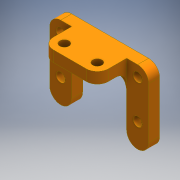
# Autodesk Inventor part: cam_holder
Saved by Autodesk Inventor 2016 (Build 200138000, 138)
## iProperties
Created: 2016-09-23
Part Number: cam_holder
Material: Nylon 6/6
Document SubType Name: Modeling
Designer: Jakub
Density: 1.13 g/cm^3
Appearance: Nylon 6
Author: Jakub
Autodesk Inventor part; units mm, degrees
ref_plane "YZ Plane" through (0, 0, 0) normal (1, 0, 0) x (0, 1, 0)
ref_plane "XZ Plane" through (0, 0, 0) normal (0, 1, 0) x (-1, 0, 0)
ref_plane "XY Plane" through (0, 0, 0) normal (0, 0, 1) x (1, 0, 0)
sketch "Sketch1" plane through (0, 0, 0) normal (0, 1, 0) x (-1, 0, 0)
  line L0 (13.5, 10) -> (-13.5, 10)
  line L1 (-13.5, 10) -> (-13.5, -10)
  line L2 (-13.5, -10) -> (13.5, -10)
  line L3 (13.5, -10) -> (13.5, 10)
  line L4 (13.5, 10) -> (-13.5, -10) construction
  line L5 (-13.5, 10) -> (13.5, -10) construction
  point P0 (0, 0)
  dimension "d0" = 27
  dimension "d1" = 20
  constraints: 12 end point, 2 midpoint, 2 parallel, 1 horizontal, 1 perpendicular
  measures "d0" distance of L2.end L1.end
  measures "d1" distance of L1.end L0.end
extrude "Extrusion1" add sketch "Sketch1" along normal blind 3
sketch "Sketch2" plane through (0, 3, 0) normal (0, 1, 0) x (1, 0, 0)
  line L0 (-13.5, -10) -> (13.5, -10) projected
  line L1 (0, -10) -> (-10.5, -10)
  line L2 (-10.5, -10) -> (-10.5, -7)
  line L3 (-10.5, -7) -> (-10.5, 3.5)
  circle A0 centre (-10.5, -7) radius 1.25
  circle A1 centre (-10.5, 3.5) radius 1.25
  line L4 (-10.5, -7) -> (10.5, -7)
  line L5 (10.5, -7) -> (10.5, 3.5)
  circle A2 centre (10.5, -7) radius 1.25
  circle A3 centre (10.5, 3.5) radius 1.25
  point P0 (0, 0)
  dimension "d4" = 10.5
  dimension "d5" = 3
  dimension "d6" = 10.5
  dimension "d7" = 2.5
  dimension "d8" = 2.5
  dimension "d9" = 21
  dimension "d10" = 10.5
  dimension "d11" = 2.5
  dimension "d12" = 2.5
  constraints: 10 end point, 4 centre point, 4 coincident, 2 point on line, 1 horizontal, 1 midpoint, 1 perpendicular, 1 vertical
  measures "d4" distance of L1.start L1.end
  measures "d5" distance of L1.end L2.end
  measures "d6" distance of L2.end L3.end
  measures "d7" diameter of A0
  measures "d8" diameter of A1
  measures "d9" distance of L4.start L4.end
  measures "d10" distance of L4.end L5.end
  measures "d11" diameter of A2
  measures "d12" diameter of A3
extrude "Extrusion2" cut sketch "Sketch2" against normal up to next
sketch "Sketch3" plane through (0, 0, 0) normal (0, -1, 0) x (1, 0, 0)
  line L0 (-13.5, 10) -> (13.5, 10) projected
  line L1 (0, 10) -> (0, 8.5)
  line L2 (7.5, 7) -> (-7.5, 7)
  line L3 (-7.5, 7) -> (-7.5, 10)
  line L4 (-7.5, 10) -> (7.5, 10)
  line L5 (7.5, 10) -> (7.5, 7)
  line L6 (7.5, 7) -> (-7.5, 10) construction
  line L7 (-7.5, 7) -> (7.5, 10) construction
  point P0 (0, 0)
  dimension "d15" = 1.5
  dimension "d16" = 15
  dimension "d17" = 3
  constraints: 14 end point, 3 midpoint, 2 parallel, 1 horizontal, 1 perpendicular, 1 vertical
  measures "d15" distance of L1.start L1.end
  measures "d16" distance of L3.end L4.end
  measures "d17" distance of L2.end L3.end
extrude "Extrusion3" add sketch "Sketch3" along normal blind 8
sketch "Sketch4" plane through (7.5, 0, 7) normal (0, 0, -1) x (-1, 0, 0)
  circle A0 centre (3, -5) radius 1.25
  circle A1 centre (12, -5) radius 1.25
  line L0 (0, 0) -> (0, -8) projected
  line L1 (15, -8) -> (0, -8) projected
  line L2 (15, 0) -> (15, -8) projected
  point P0 (7.5, 0)
  dimension "d20" = 2.5
  dimension "d21" = 2.5
  dimension "d22" = 3
  dimension "d23" = 3
  dimension "d24" = 3
  dimension "d25" = 3
  constraints: 2 centre point
  measures "d20" diameter of A0
  measures "d21" diameter of A1
  measures "d22" distance from line of L0 A0.centre
  measures "d23" distance from line of L1 A0.centre
  measures "d24" distance from line of L2 A1.centre
  measures "d25" distance from line of L1 A1.centre
extrude "Extrusion4" cut sketch "Sketch4" against normal up to next
sketch "Sketch5" plane through (0, 0, 0) normal (0, -1, 0) x (1, 0, 0)
  line L0 (13.5, -10) -> (-13.5, -10) projected
  line L1 (13.5, -10) -> (7.5, -10)
  line L2 (7.5, -10) -> (-7.5, -10)
  line L3 (-7.5, -10) -> (-7.5, 7)
  line L4 (-7.5, 7) -> (7.5, 7)
  line L5 (7.5, 7) -> (7.5, -10)
  point P0 (0, 0)
  dimension "d28" = 6
  constraints: 10 end point, 2 parallel, 1 horizontal, 1 perpendicular, 1 point on line
  measures "d28" distance of L0.start L1.end
extrude "Extrusion5" cut sketch "Sketch5" against normal up to next
fillet "Fillet1" radius 5 2 edges at (-7.5, 1.5, 7) (7.5, 1.5, 7)
fillet "Fillet2" radius 3 10 edges at (7.5, 1.5, -10) (13.5, 1.5, -10) (-7.5, 1.5, -10) (-13.5, 1.5, -10) (-13.5, 1.5, 10) (13.5, 1.5, 10) (-7.5, -8, 8.5) (7.5, -8, 8.5) (-5, 0, 7) (5, 0, 7)
body "Solid1"
